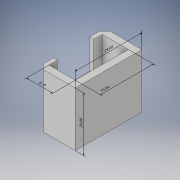
# Autodesk Inventor part: Connect_Female_Beauty
Saved by Autodesk Inventor 2019 (Build 230136000, 136)
## iProperties
Created: 2020-03-29
Part Number: Connect_Female_Beauty
Material: Generico
Document SubType Name: Modeling
Designer: Administrator
Density: 1 g/cm^3
Appearance: Default
Author: Administrator
Autodesk Inventor part; units mm, degrees
ref_plane "YZ Plane" through (0, 0, 0) normal (1, 0, 0) x (0, 1, 0)
ref_plane "XZ Plane" through (0, 0, 0) normal (0, 1, 0) x (-1, 0, 0)
ref_plane "XY Plane" through (0, 0, 0) normal (0, 0, 1) x (1, 0, 0)
sketch "Sketch1" plane through (0, 0, 0) normal (0, 1, 0) x (-1, 0, 0)
  line L0 (-7.35, 12.3) -> (7.35, 12.3)
  line L1 (7.35, 12.3) -> (7.35, -12.3)
  line L2 (7.35, -12.3) -> (-7.35, -12.3)
  line L3 (-7.35, -12.3) -> (-7.35, 12.3)
  line L4 (-7.35, 12.3) -> (7.35, -12.3) construction
  line L5 (7.35, 12.3) -> (-7.35, -12.3) construction
  point P0 (0, 0)
  dimension "d0" = 14.7
  dimension "d1" = 24.6
  constraints: 12 end point, 2 midpoint, 2 parallel, 1 horizontal, 1 perpendicular
  measures "d0" distance of L1.end L2.end
  measures "d1" distance of L0.end L1.end
extrude "Extrusion1" add sketch "Sketch1" along normal blind 20
sketch "Sketch2" plane through (0, 20, 0) normal (0, 1, 0) x (1, 0, 0)
  line L0 (4.85, -9.8) -> (-4.85, -9.8)
  line L1 (-4.85, -9.8) -> (-4.85, 9.8)
  line L2 (-4.85, 9.8) -> (4.85, 9.8)
  line L3 (4.85, 9.8) -> (4.85, -9.8)
  line L4 (4.85, -9.8) -> (-4.85, 9.8) construction
  line L5 (-4.85, -9.8) -> (4.85, 9.8) construction
  point P0 (0, 0)
  point P1 (-6.1069, 0)
  dimension "d4" = 9.7
  dimension "d5" = 19.6
  constraints: 12 end point, 2 midpoint, 2 parallel, 1 horizontal, 1 perpendicular
  measures "d4" distance of L1.end L2.end
  measures "d5" distance of L0.end L1.end
extrude "Extrusion2" cut sketch "Sketch2" against normal blind 17.5
sketch "Sketch3" plane through (-7.35, 0, -12.3) normal (-1, 0, 0) x (0, 0, 1)
  point P0 (12.3, 0)
sketch "Sketch4" plane through (0, 20, 0) normal (0, 1, 0) x (1, 0, 0)
  line L0 (-4.85, -9.8) -> (-4.85, 9.8) projected
  line L1 (-7.35, 12.3) -> (-7.35, -12.3) projected
  line L2 (-4.85, -6.65) -> (-7.35, -6.65)
  line L3 (-7.35, -6.65) -> (-7.35, 6.65)
  line L4 (-7.35, 6.65) -> (-4.85, 6.65)
  line L5 (-4.85, 6.65) -> (-4.85, -6.65)
  line L6 (-4.85, -6.65) -> (-7.35, 6.65) construction
  line L7 (-7.35, -6.65) -> (-4.85, 6.65) construction
  point P0 (0, 0)
  point P1 (-6.1, 0)
  dimension "d8" = 13.3
  constraints: 12 end point, 2 midpoint, 2 parallel, 1 horizontal, 1 perpendicular, 1 point on line
  measures "d8" distance of L2.end L3.end
extrude "Extrusion3" cut sketch "Sketch4" against normal blind 11
move faces "Move1" translate (1, 0, 0) faces at (-7.35, 3, 2.2167)
chamfer "Chamfer1" distance 2 angle 45 3 edges at (-6.35, 0, 0) (-6.35, 10, 12.3) (-6.35, 10, -12.3)
body "Solid1"
